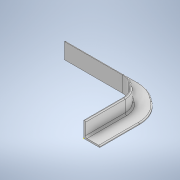
# Autodesk Inventor part: lab_4_3
Saved by Autodesk Inventor 2020 (Build 240168000, 168)
## iProperties
Created: 2020-03-31
Part Number: lab_4_3
Material: Типовые
Document SubType Name: Modeling
Designer: User
Density: 1 g/cm^3
Appearance: По умолчанию
Author: User
Autodesk Inventor part; units mm, degrees
ref_plane "YZ Plane" through (0, 0, 0) normal (1, 0, 0) x (0, 1, 0)
ref_plane "XZ Plane" through (0, 0, 0) normal (0, 1, 0) x (-1, 0, 0)
ref_plane "XY Plane" through (0, 0, 0) normal (0, 0, 1) x (1, 0, 0)
sketch "Эскиз1" plane through (0, 0, 0) normal (0, 0, 1) x (1, 0, 0)
  line L0 (0, 0) -> (0, 50)
  line L1 (0, 50) -> (2, 50)
  line L2 (5, 47) -> (5, 10)
  line L3 (10, 5) -> (47, 5)
  line L4 (50, 2) -> (50, 0)
  line L5 (50, 0) -> (0, 0)
  arc A0 (5, 47) -> (2, 50) centre (2, 47) ccw
  arc A1 (5, 10) -> (10, 5) centre (10, 10) ccw
  arc A2 (50, 2) -> (47, 5) centre (47, 2) ccw
  point P0 (5, 50)
  point P1 (5, 5)
  point P2 (50, 5)
  dimension "d6" = 50
  dimension "d7" = 5
  dimension "d8" = 45
  dimension "d9" = 45
  dimension "d10" = 3
  dimension "d11" = 5
  dimension "d12" = 3
  constraints: 12 end point, 6 point on circle, 6 point on line, 6 tangent, 5 perpendicular, 3 centre point, 1 vertical
  measures "d6" distance of L0.start L0.end
  measures "d7" distance of L0.end point (5, 50)
  measures "d8" distance of point (5, 50) point (5, 5)
  measures "d9" distance of point (5, 5) point (50, 5)
  measures "d10" radius of A0
  measures "d11" radius of A1
  measures "d12" radius of A2
sketch "Эскиз2" plane through (0, 0, 0) normal (0, 1, 0) x (-1, 0, 0)
  point P0 (0, 0)
sketch "Эскиз3" plane through (0, 0, 0) normal (0, 1, 0) x (-1, 0, 0)
  line L0 (0, 0) -> (0, -125.202)
  line L1 (19.7417, -165.0069) -> (32.6025, -174.7832)
  line L2 (62.8608, -184.9783) -> (246.0141, -184.9783)
  arc A0 (0, -125.202) -> (19.7417, -165.0069) centre (50, -125.202) ccw
  arc A1 (32.6025, -174.7832) -> (62.8608, -184.9783) centre (62.8608, -134.9783) ccw
  point P0 (0, -150)
  point P1 (46.0141, -184.9783)
  dimension "d13" = 150
  dimension "d14" = 200
  dimension "d15" = 50
  constraints: 6 end point, 4 point on circle, 4 point on line, 4 tangent, 2 centre point, 1 equal radius, 1 perpendicular, 1 vertical
  measures "d13" distance of L0.start point (0, -150)
  measures "d14" distance of point (46.014, -184.978) L2.end
  measures "d15" radius of A0
sweep "Сдвиг1" add profiles "Эскиз1" path "Эскиз3"
